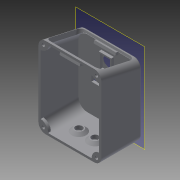
# Autodesk Inventor part: obudowa - budzik v3 dol
Saved by Autodesk Inventor 2014 (Build 180170000, 170)
## iProperties
Created: 2018-03-05
Part Number: obudowa - budzik v3 dol
Material: Generic
Document SubType Name: Modeling
Designer: HP820
Density: 1 g/cm^3
Appearance: Default
Author: HP820
Autodesk Inventor part; units mm, degrees
ref_plane "YZ Plane" through (0, 0, 0) normal (1, 0, 0) x (0, 1, 0)
ref_plane "XY Plane" through (0, 0, 0) normal (0, 0, 1) x (1, 0, 0)
sketch "Sketch1" plane through (0, 0, 0) normal (0, 1, 0) x (-1, 0, 0)
  line L0 (-35, 45) -> (35, 45)
  line L1 (35, 45) -> (35, -45)
  line L2 (35, -45) -> (-35, -45)
  line L3 (-35, -45) -> (-35, 45)
  line L4 (-35, 45) -> (35, -45) construction
  line L5 (35, 45) -> (-35, -45) construction
  point P0 (0, 0)
  dimension "d0" = 70
  dimension "d1" = 90
  constraints: 12 end point, 2 midpoint, 2 parallel, 1 horizontal, 1 perpendicular
  measures "d0" distance of L1.end L2.end
  measures "d1" distance of L0.end L1.end
ref_plane "Work Plane1" through (0, 45, 0) normal (0, 1, 0) x (-1, 0, 0)
sketch "Sketch2" plane through (0, 45, 0) normal (0, 1, 0) x (-1, 0, 0)
  line L0 (35, -45) -> (-35, -45)
  line L1 (-35, -45) -> (-35, 35)
  line L2 (-35, 35) -> (35, 35)
  line L3 (35, 35) -> (35, -45)
  point P0 (0, 0)
  dimension "d3" = 80
  constraints: 8 end point, 2 parallel, 1 horizontal, 1 perpendicular
  measures "d3" distance of L0.end L1.end
loft "Loft1" add profiles "Sketch1", "Sketch2"
sketch "Sketch3" plane through (-35, 0, 45) normal (0, 0.2169305, 0.9761871) x (1, 0, 0)
  line L0 (5, 43.0489) -> (65, 43.0489)
  line L1 (65, 43.0489) -> (65, 3.0489)
  line L2 (65, 3.0489) -> (5, 3.0489)
  line L3 (5, 3.0489) -> (5, 43.0489)
  line L4 (5, 43.0489) -> (65, 3.0489) construction
  line L5 (65, 43.0489) -> (5, 3.0489) construction
  point P0 (35, 9.7619)
  point P1 (35, 23.0489)
  dimension "d8" = 60
  dimension "d9" = 40
  constraints: 12 end point, 2 midpoint, 2 parallel, 1 horizontal, 1 perpendicular
  measures "d8" distance of L1.end L2.end
  measures "d9" distance of L0.end L1.end
sketch "Sketch4" plane through (-35, 0, 45) normal (0, -1, 0) x (1, 0, 0)
  line L0 (2.5, -2.5) -> (67.5, -2.5)
  line L1 (67.5, -2.5) -> (67.5, -87.5)
  line L2 (67.5, -87.5) -> (2.5, -87.5)
  line L3 (2.5, -87.5) -> (2.5, -2.5)
  line L4 (2.5, -2.5) -> (67.5, -87.5) construction
  line L5 (67.5, -2.5) -> (2.5, -87.5) construction
  point P0 (35, -45)
  dimension "d10" = 65
  dimension "d11" = 85
  constraints: 12 end point, 2 midpoint, 2 parallel, 1 horizontal, 1 perpendicular
  measures "d10" distance of L1.end L2.end
  measures "d11" distance of L0.end L1.end
sketch "Sketch5" plane through (-35, 45, 35) normal (0, 1, 0) x (1, 0, 0)
  line L0 (2.5, 2.5) -> (67.5, 2.5)
  line L1 (67.5, 2.5) -> (67.5, 77.5)
  line L2 (67.5, 77.5) -> (2.5, 77.5)
  line L3 (2.5, 77.5) -> (2.5, 2.5)
  line L4 (2.5, 2.5) -> (67.5, 77.5) construction
  line L5 (67.5, 2.5) -> (2.5, 77.5) construction
  point P0 (35, 35)
  point P1 (35, 40)
  dimension "d12" = 65
  dimension "d13" = 75
  constraints: 12 end point, 2 midpoint, 2 parallel, 1 horizontal, 1 perpendicular
  measures "d12" distance of L2.end L1.end
  measures "d13" distance of L1.end L0.end
extrude "Extrusion1" cut sketch "Sketch3" against normal blind 5
fillet "Fillet1" radius 5 4 edges at (-30, 41.4812, 33.2199) (-30, 2.4337, 41.8972) (30, 41.4812, 33.2199) (30, 2.4337, 41.8972)
loft "Loft2" cut profiles "Sketch5", "Sketch4"
sketch "Sketch6" plane through (32.5, 45, 32.5) normal (0, -0.2169305, -0.9761871) x (-1, 0, 0)
  line L0 (7.5, -43.5912) -> (57.5, -43.5912) projected
  line L1 (57.5, -3.5912) -> (7.5, -3.5912) projected
  line L2 (21.2702, -45.7222) -> (43.7298, -45.7222)
  line L3 (43.7298, -45.7222) -> (43.7298, -41.4601)
  line L4 (43.7298, -41.4601) -> (21.2702, -41.4601)
  line L5 (21.2702, -41.4601) -> (21.2702, -45.7222)
  line L6 (21.2702, -45.7222) -> (43.7298, -41.4601) construction
  line L7 (43.7298, -45.7222) -> (21.2702, -41.4601) construction
  line L8 (20.4275, -5.9981) -> (44.5725, -5.9981)
  line L9 (44.5725, -5.9981) -> (44.5725, -1.1843)
  line L10 (44.5725, -1.1843) -> (20.4275, -1.1843)
  line L11 (20.4275, -1.1843) -> (20.4275, -5.9981)
  line L12 (20.4275, -5.9981) -> (44.5725, -1.1843) construction
  line L13 (44.5725, -5.9981) -> (20.4275, -1.1843) construction
  point P0 (32.5, -36.8782)
  point P1 (32.5, -43.5912)
  point P2 (32.5, -3.5912)
  constraints: 24 end point, 6 midpoint, 4 parallel, 2 horizontal, 2 perpendicular
extrude "Extrusion2" add sketch "Sketch6" along normal blind 3
fillet "Fillet2" radius 8 4 edges at (35, 22.5, 40) (-35, 22.5, 40) (35, 22.5, -45) (-35, 22.5, -45)
fillet "Fillet3" radius 10 4 edges at (32.5, 22.5, 37.5) (32.5, 22.5, -42.5) (-32.5, 22.5, 37.5) (-32.5, 22.5, -42.5)
sketch "Sketch7" plane through (-27, 45, 35) normal (0, 1, 0) x (1, 0, 0)
  arc A0 (0, 80) -> (-8, 72) centre (0, 72) ccw projected
  line L0 (49.5, 2.5) -> (4.5, 2.5) projected
  ellipse E0 centre (4.5, 12.7439) end of major axis (4.5, 2.5) minor radius 10 (-5.5, 12.7439) -> (4.5, 2.5) ccw projected
  line L1 (-5.5, 12.7439) -> (-5.5, 67.5) projected
  arc A1 (4.5, 77.5) -> (-5.5, 67.5) centre (4.5, 67.5) ccw projected
  line L2 (4.5, 77.5) -> (49.5, 77.5) projected
  arc A2 (59.5, 67.5) -> (49.5, 77.5) centre (49.5, 67.5) ccw projected
  line L3 (59.5, 67.5) -> (59.5, 12.7439) projected
  ellipse E1 centre (49.5, 12.7439) end of major axis (49.5, 2.5) minor radius 10 (49.5, 2.5) -> (59.5, 12.7439) ccw projected
  arc A3 (0, 80) -> (-8, 72) centre (0, 72) ccw projected
  line L4 (-8, 8.1952) -> (-8, 72) projected
  ellipse E2 centre (0, 8.1952) end of major axis (0, 0) minor radius 8 (-8, 8.1952) -> (0, 0) ccw projected
  line L5 (54, 0) -> (0, 0) projected
  ellipse E3 centre (54, 8.1952) end of major axis (54, 0) minor radius 8 (54, 0) -> (62, 8.1952) ccw projected
  line L6 (62, 72) -> (62, 8.1952) projected
  arc A4 (62, 72) -> (54, 80) centre (54, 72) ccw projected
  line L7 (0, 80) -> (54, 80) projected
  line L8 (49.5, 2.5) -> (4.5, 2.5) projected
  ellipse E4 centre (4.5, 12.7439) end of major axis (4.5, 2.5) minor radius 10 (-5.5, 12.7439) -> (4.5, 2.5) ccw projected
  line L9 (-5.5, 12.7439) -> (-5.5, 67.5) projected
  arc A5 (4.5, 77.5) -> (-5.5, 67.5) centre (4.5, 67.5) ccw projected
  line L10 (4.5, 77.5) -> (49.5, 77.5) projected
  arc A6 (59.5, 67.5) -> (49.5, 77.5) centre (49.5, 67.5) ccw projected
  line L11 (59.5, 67.5) -> (59.5, 12.7439) projected
  ellipse E5 centre (49.5, 12.7439) end of major axis (49.5, 2.5) minor radius 10 (49.5, 2.5) -> (59.5, 12.7439) ccw projected
  point P0 (27, 35)
  constraints: 6 other
extrude "Extrusion3" add sketch "Sketch7" against normal blind 3 contours L0 E0 L1 A1 L2 A2 L3 E1
fillet "Fillet4" radius 2 8 edges at (-32.6569, 45, 32.5997) (-35, 45, -5.0976) (-32.6569, 45, -42.6569) (0, 45, -45) (32.6569, 45, -42.6569) (35, 45, -5.0976) (32.6569, 45, 32.5997) (0, 45, 35)
sketch "Sketch8" plane through (-27, 45, 33.3957) normal (0, 1, 0) x (1, 0, 0)
  circle A0 centre (27, 61.879) radius 4.75
  point P0 (27, 33.3957)
  dimension "d28" = 9.5
  constraints: 1 centre point
  measures "d28" diameter of A0
extrude "Extrusion4" cut sketch "Sketch8" against normal blind 3
sketch "Sketch9" plane through (-27, 45, 33.3957) normal (0, 1, 0) x (1, 0, 0)
  line L0 (49.5, 0.8957) -> (4.5, 0.8957) projected
  line L1 (60, 70.3957) -> (60, 6.1464) projected
  line L2 (-6, 6.1464) -> (-6, 70.3957) projected
  line L3 (9, 44.1757) -> (20, 44.1757)
  line L4 (20, 44.1757) -> (20, 38.1757)
  line L5 (20, 38.1757) -> (9, 38.1757)
  line L6 (9, 38.1757) -> (9, 44.1757)
  line L7 (9, 44.1757) -> (20, 38.1757) construction
  line L8 (20, 44.1757) -> (9, 38.1757) construction
  line L9 (34, 44.1757) -> (45, 44.1757)
  line L10 (45, 44.1757) -> (45, 38.1757)
  line L11 (45, 38.1757) -> (34, 38.1757)
  line L12 (34, 38.1757) -> (34, 44.1757)
  line L13 (34, 44.1757) -> (45, 38.1757) construction
  line L14 (45, 44.1757) -> (34, 38.1757) construction
  point P0 (27, 33.3957)
  point P1 (14.5, 41.1757)
  point P2 (39.5, 41.1757)
  dimension "d31" = 11
  dimension "d32" = 6
  dimension "d33" = 11
  dimension "d34" = 6
  dimension "d35" = 15
  dimension "d36" = 15
  dimension "d37" = 37.28
  constraints: 24 end point, 4 midpoint, 4 parallel, 2 horizontal, 2 perpendicular
  measures "d31" distance of L4.end L5.end
  measures "d32" distance of L3.end L4.end
  measures "d33" distance of L10.end L11.end
  measures "d34" distance of L9.end L10.end
  measures "d35" distance between parallel lines of L2 L6
  measures "d36" distance between parallel lines of L1 L10
  measures "d37" distance between parallel lines of L5 L0
extrude "Extrusion5" cut sketch "Sketch9" against normal blind 3
sketch "Sketch10" plane through (-27, 45, 33.3957) normal (0, 1, 0) x (1, 0, 0)
  circle A0 centre (27, 15.8957) radius 5
  line L0 (49.5, 0.8957) -> (4.5, 0.8957) projected
  point P0 (27, 33.3957)
  dimension "d40" = 10
  dimension "d43" = 15
  constraints: 1 centre point
  measures "d40" diameter of A0
  measures "d43" distance from line of A0.centre L0
extrude "Extrusion6" cut sketch "Sketch10" against normal blind 3
chamfer "Chamfer1" distance 3 angle 45 1 edges at (-5, 45, 17.5)
fillet "Fillet5" radius 3 1 edges at (-7.9999, 45, 17.5)
sketch "Sketch11" plane through (-27, 0, -45) normal (0, -1, 0) x (1, 0, 0)
  ellipse E0 centre (49.5, 77.2561) end of major axis (49.5, 87.5) minor radius 10 (59.5, 77.2561) -> (49.5, 87.5) ccw projected
  ellipse E1 centre (4.5, 77.2561) end of major axis (4.5, 87.5) minor radius 10 (4.5, 87.5) -> (-5.5, 77.2561) ccw projected
  arc A0 (-8, 8) -> (0, 0) centre (0, 8) ccw projected
  line L0 (0, 0) -> (54, 0) projected
  arc A1 (54, 0) -> (62, 8) centre (54, 8) ccw projected
  line L1 (62, 8) -> (62, 81.8048) projected
  ellipse E2 centre (54, 81.8048) end of major axis (54, 90) minor radius 8 (62, 81.8048) -> (54, 90) ccw projected
  ellipse E3 centre (0, 81.8048) end of major axis (0, 90) minor radius 8 (0, 90) -> (-8, 81.8048) ccw projected
  line L2 (-8, 81.8048) -> (-8, 8) projected
  arc A2 (2.1949, 0) -> (-8, 11.8728) centre (-6.2764, 3.0394) ccw
  arc A3 (62, 11.8728) -> (51.8051, 0) centre (60.2764, 3.0394) ccw
  arc A4 (50.6584, 87.431) -> (59.4132, 78.603) centre (59.6569, 87.5997) ccw
  arc A5 (-5.4132, 78.603) -> (3.3416, 87.431) centre (-5.6569, 87.5997) ccw
  point P0 (27, 45)
  dimension "d48" = 18
  dimension "d49" = 18
  dimension "d50" = 18
  dimension "d51" = 18
  constraints: 10 point on circle, 4 centre point, 4 point on line, 10 other
  measures "d48" diameter of A2
  measures "d49" diameter of A3
  measures "d50" diameter of A4
  measures "d51" diameter of A5
extrude "Extrusion7" add sketch "Sketch11" against normal blind 3
sketch "Sketch12" plane through (-27, 0, 45) normal (0, -1, 0) x (1, 0, 0)
  line L0 (-2.5808, -84.6651) -> (56.5808, -84.6651)
  line L1 (56.5808, -84.6651) -> (56.5808, -5.3349)
  line L2 (56.5808, -5.3349) -> (-2.5808, -5.3349)
  line L3 (-2.5808, -5.3349) -> (-2.5808, -84.6651)
  line L4 (-2.5808, -84.6651) -> (56.5808, -5.3349) construction
  line L5 (56.5808, -84.6651) -> (-2.5808, -5.3349) construction
  circle A0 centre (-2.5808, -5.3349) radius 1.25
  circle A1 centre (56.5808, -5.3349) radius 1.25
  circle A2 centre (56.5808, -84.6651) radius 1.25
  circle A3 centre (-2.5808, -84.6651) radius 1.25
  point P0 (27, -45)
  dimension "d54" = 2.5
  dimension "d55" = 2.5
  dimension "d56" = 2.5
  dimension "d57" = 2.5
  constraints: 12 end point, 4 centre point, 4 coincident, 2 midpoint, 2 parallel, 1 horizontal, 1 perpendicular
  measures "d54" diameter of A0
  measures "d55" diameter of A1
  measures "d56" diameter of A2
  measures "d57" diameter of A3
extrude "Extrusion8" cut sketch "Sketch12" against normal blind 3 contours L3 A3 L0 | L0 A3 L3 | A2 L1 L0 | L0 L1 A2 | A0 L2 L3 | L3 L2 A0 | A1 L2 L1 | L1 L2 A1
chamfer "Chamfer2" distance 0.5 angle 45 4 edges at (28.3308, 0, 39.6651) (-30.8308, 0, 39.6651) (-30.8308, 0, -39.6651) (28.3308, 0, -39.6651)
sketch "Sketch14" plane through (-27, 42, 35) normal (0, -1, 0) x (1, 0, 0)
  circle A0 centre (27, -17.5) radius 5 projected
  line L0 (21.5, -11) -> (32.5, -11)
  line L1 (32.5, -11) -> (32.5, -24)
  line L2 (32.5, -24) -> (21.5, -24)
  line L3 (21.5, -24) -> (21.5, -11)
  line L4 (21.5, -11) -> (32.5, -24) construction
  line L5 (32.5, -11) -> (21.5, -24) construction
  line L6 (21.5, -24) -> (32.5, -24)
  line L7 (32.5, -24) -> (32.5, -26)
  line L8 (32.5, -26) -> (21.5, -26)
  line L9 (21.5, -26) -> (21.5, -24)
  line L10 (20, -9.5) -> (34, -9.5)
  line L11 (34, -9.5) -> (34, -27.5)
  line L12 (34, -27.5) -> (20, -27.5)
  line L13 (20, -27.5) -> (20, -9.5)
  point P0 (27, -35)
  dimension "d69" = 11
  dimension "d70" = 13
  dimension "d71" = 2
  dimension "d72" = 1.5
  dimension "d73" = 1.5
  dimension "d74" = 1.5
  dimension "d75" = 1.5
  constraints: 28 end point, 6 parallel, 3 horizontal, 3 perpendicular, 2 midpoint
  measures "d69" distance of L1.end L2.end
  measures "d70" distance of L0.end L1.end
  measures "d71" distance of L6.end L7.end
  measures "d72" distance between parallel lines of L3 L13
  measures "d73" distance between parallel lines of L12 L8
  measures "d74" distance between parallel lines of L10 L0
  measures "d75" distance between parallel lines of L11 L1
extrude "Extrusion10" add sketch "Sketch14" along normal blind 3 contours L10 L11 L12 L13
sketch "Sketch15" plane through (27, 0, -45) normal (0, 0, -1) x (-1, 0, 0)
  line L0 (0, 0) -> (0, 43) projected
  line L1 (54, 0) -> (0, 0) projected
  line L2 (54, 43) -> (54, 0) projected
  circle A0 centre (18, 19) radius 3.75
  circle A1 centre (36, 19) radius 3.75
  point P0 (27, 0)
  dimension "d78" = 7.5
  dimension "d79" = 7.5
  dimension "d80" = 19
  dimension "d81" = 19
  dimension "d82" = 18
  dimension "d83" = 18
  constraints: 2 centre point
  measures "d78" diameter of A0
  measures "d79" diameter of A1
  measures "d80" distance from line of L1 A0.centre
  measures "d81" distance from line of L1 A1.centre
  measures "d82" distance from line of L0 A0.centre
  measures "d83" distance from line of L2 A1.centre
extrude "Extrusion11" cut sketch "Sketch15" against normal blind 3
fillet "Fillet6" radius 2 2 edges at (-5.25, 19, -45) (12.75, 19, -45)
sketch "Sketch16" plane through (-22.5, 0, -42.5) normal (0, 0, 1) x (1, 0, 0)
  circle A0 centre (31.5, 19) radius 3.75 projected
  circle A1 centre (13.5, 19) radius 3.75 projected
  circle A2 centre (13.5, 19) radius 5
  circle A3 centre (31.5, 19) radius 5
  point P0 (22.5, 0)
  dimension "d87" = 10
  dimension "d88" = 10
  constraints: 2 centre point, 2 coincident
  measures "d87" diameter of A2
  measures "d88" diameter of A3
extrude "Extrusion12" add sketch "Sketch16" along normal blind 3
chamfer "Chamfer3" distance 3 angle 45 2 edges at (-14, 19, -42.5) (4, 19, -42.5)
body "Solid1"
